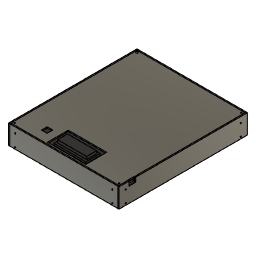
Case (Autodesk Fusion 360 design; units mm, degrees)
Autodesk Fusion 360 part; units mm, degrees
sketch "Sketch1" plane through (0, 0, 0) normal (0, 0, 1) x (1, 0, 0) in component "PCB"
  line L0 (-131, 153.5) -> (131, 153.5) construction
  line L1 (131, 153.5) -> (131, -153.5) construction
  line L2 (131, -153.5) -> (-131, -153.5) construction
  line L3 (-131, -153.5) -> (-131, 153.5) construction
  line L4 (-131, 153.5) -> (131, -153.5) construction
  line L5 (131, 153.5) -> (-131, -153.5) construction
  line L6 (-135, 157.5) -> (135, 157.5)
  line L7 (135, 157.5) -> (135, -157.5)
  line L8 (135, -157.5) -> (-135, -157.5)
  line L9 (-135, -157.5) -> (-135, 157.5)
  line L10 (-135, 157.5) -> (135, -157.5) construction
  line L11 (135, 157.5) -> (-135, -157.5) construction
  circle A0 centre (-131, 153.5) radius 1.6
  circle A1 centre (131, 153.5) radius 1.6
  circle A2 centre (-131, -153.5) radius 1.6
  circle A3 centre (131, -153.5) radius 1.6
  line L12 (135, -127.52) -> (128, -127.52) construction
  line L13 (128, -127.52) -> (128, -123.02)
  line L14 (128, -123.02) -> (135, -123.02)
  line L15 (128, -132.02) -> (135, -132.02)
  line L16 (128, -127.52) -> (128, -132.02)
  line L17 (122.64, -122.688) -> (112.36, -122.688)
  line L18 (112.36, -122.688) -> (112.36, -120.028)
  line L19 (112.36, -120.028) -> (122.64, -120.028)
  line L20 (122.64, -120.028) -> (122.64, -122.688)
  line L21 (122.64, -122.688) -> (112.36, -120.028) construction
  line L22 (112.36, -122.688) -> (122.64, -120.028) construction
  circle A4 centre (113.69, -121.358) radius 0.5
  circle A5 centre (116.23, -121.358) radius 0.5
  circle A6 centre (118.77, -121.358) radius 0.5
  circle A7 centre (121.31, -121.358) radius 0.5
  line L23 (113.69, -121.358) -> (116.23, -121.358) construction
  line L24 (116.23, -121.358) -> (118.77, -121.358) construction
  line L25 (118.77, -121.358) -> (121.31, -121.358) construction
  line L26 (121.31, -121.358) -> (122.64, -121.358) construction
  line L27 (113.69, -121.358) -> (112.36, -121.358) construction
  line L28 (-40.14, -109.718) -> (40.14, -109.718)
  line L29 (40.14, -109.718) -> (40.14, -145.998)
  line L30 (40.14, -145.998) -> (-40.14, -145.998)
  line L31 (-40.14, -145.998) -> (-40.14, -109.718)
  line L32 (-40.14, -109.718) -> (40.14, -145.998) construction
  line L33 (40.14, -109.718) -> (-40.14, -145.998) construction
  line L34 (-36.5, -115.358) -> (36.5, -115.358)
  line L35 (36.5, -115.358) -> (36.5, -140.358)
  line L36 (36.5, -140.358) -> (-36.5, -140.358)
  line L37 (-36.5, -140.358) -> (-36.5, -115.358)
  line L38 (-36.5, -115.358) -> (36.5, -140.358) construction
  line L39 (36.5, -115.358) -> (-36.5, -140.358) construction
  point P0 (117.5, -121.358)
  point P1 (0, -127.858)
  point P2 (0, -127.858)
  dimension "d1" = 262
  dimension "d2" = 307
  dimension "d3" = 270
  dimension "d4" = 315
  dimension "d5" = 3.2
  dimension "d8" = 29.98
  dimension "d9" = 9
  dimension "d10" = 7
  dimension "d17" = 10.28
  dimension "d18" = 2.66
  dimension "d19" = 2.54
  dimension "d20" = 1
  dimension "d21" = 36.142
  dimension "d22" = 17.5
  dimension "d30" = 29.642
  dimension "d31" = 135
  dimension "d32" = 80.28
  dimension "d33" = 36.28
  dimension "d34" = 73
  dimension "d35" = 25
  constraint horizontal L0
  constraint perpendicular L0 L1
  constraint parallel L0 L2
  constraint parallel L1 L3
  constraint coincident L4 origin
  constraint coincident L5 origin
  constraint horizontal L6
  constraint perpendicular L6 L7
  constraint parallel L6 L8
  constraint parallel L7 L9
  constraint coincident L10 origin
  constraint coincident L11 origin
  constraint coincident L0.start L3.end
  constraint coincident L0.end L1.start
  constraint coincident L2.end L3.start
  constraint coincident L1.end L2.start
  constraint equal A1 A3
  constraint equal A2 A3
  constraint equal A0 A2
  constraint coincident L7 L12.start
  constraint perpendicular L1 L12
  constraint perpendicular L12 L13
  constraint coincident L7 L14.end
  constraint perpendicular L7 L14
  constraint symmetric L13.start L12 L16.start
  constraint symmetric L12 L13.end L15.start
  constraint symmetric L12 L14.end L15.end
  constraint horizontal L17
  constraint perpendicular L17 L18
  constraint parallel L17 L19
  constraint parallel L18 L20
  constraint coincident L21 P0
  constraint coincident L22 P0
  constraint coincident A4.centre L23.start
  constraint horizontal L23
  constraint coincident A5.centre L23.end
  constraint equal A4 A5
  constraint equal A5 A6
  constraint equal A6 A7
  constraint parallel L23 L24
  constraint parallel L23 L25
  constraint parallel L25 L26
  constraint coincident A6.centre L24.end
  constraint coincident A7.centre L25.end
  constraint equal L23 L24
  constraint equal L24 L25
  constraint parallel L23 L27
  constraint equal L26 L27
  constraint midpoint L18 L27.end
  constraint midpoint L20 L26.end
  constraint horizontal L28
  constraint perpendicular L28 L29
  constraint parallel L28 L30
  constraint parallel L29 L31
  constraint coincident L32 P2
  constraint coincident L33 P2
  constraint horizontal L34
  constraint perpendicular L34 L35
  constraint parallel L34 L36
  constraint parallel L35 L37
  constraint coincident L38 P2
  constraint coincident L39 P2
  constraint coincident P2 P1
  measures "d1" distance of L1.end L2.end
  measures "d2" distance of L0.end L1.end
  measures "d3" distance of L7.end L8.end
  measures "d4" distance of L6.end L7.end
  measures "d5" diameter of A0
  measures "d8" distance of L7.end L12.start
  measures "d9" distance of L14 L15
  measures "d10" distance of L13.end L14.end
  measures "d17" distance of L18.end L19.end
  measures "d18" distance of L17.end L18.end
  measures "d19" distance of A4.centre A5.centre
  measures "d20" diameter of A7
  measures "d21" distance of L8 P0
  measures "d22" distance of L7 P0
  measures "d30" distance of L8 P2
  measures "d31" distance of L9 P2
  measures "d32" distance of L28.start L28.end
  measures "d33" distance of L28.end L29.end
  measures "d34" distance of L35.end L36.end
  measures "d35" distance of L34.end L35.end
extrude "Extrude1" add sketch "Sketch1" along normal blind 1.6 contours L6 L7 L8 L9 L13 L14 L15 L16 makes body 1 in component "PCB"
extrude "Extrude2" add sketch "Sketch1" along normal blind 5 contours L7 L13 L14 L15 L16 bodies 1 in component "PCB"
extrude "Extrude3" add sketch "Sketch1" along normal blind 6.2 contours L28 L29 L30 L31 bodies 1 in component "PCB"
extrude "Extrude4" add sketch "Sketch1" along normal blind 13.15 contours L34 L35 L36 L37 bodies 1 in component "PCB"
sketch "Sketch1 (2)" plane through (0, 0, 0) normal (0, 0, 1) x (1, 0, 0) in component "Corner"
  circle A0 centre (0, 0) radius 2.3
  line L0 (0, 0) -> (0, -9.2) construction
  line L1 (0, 0) -> (9.2, 0) construction
  circle A1 centre (0, -9.2) radius 2.3
  circle A2 centre (9.2, 0) radius 2.3
  line L2 (-4.6, 4.6) -> (-4.6, -13.8)
  line L3 (-4.6, -13.8) -> (4.6, -13.8)
  line L4 (4.6, -13.8) -> (4.6, -4.6)
  line L5 (4.6, -4.6) -> (13.8, -4.6)
  line L6 (13.8, -4.6) -> (13.8, 4.6)
  line L7 (13.8, 4.6) -> (-4.6, 4.6)
  line L8 (4.6, 0) -> (4.6, 4.6) construction
  line L9 (4.6, 0) -> (4.6, -4.6) construction
  line L10 (0, -4.6) -> (4.6, -4.6) construction
  line L11 (0, -4.6) -> (-4.6, -4.6) construction
  line L12 (9.2, 0) -> (13.8, 0) construction
  line L13 (0, -9.2) -> (0, -13.8) construction
  dimension "d41" = 4.6
  dimension "d42" = 9.2
  dimension "d43" = 4.6
  dimension "d44" = 4.6
  constraint coincident A0.centre L0.start
  constraint vertical L0
  constraint perpendicular L0 L1
  constraint equal L0 L1
  constraint coincident L0.end A1.centre
  constraint coincident L1.end A2.centre
  constraint equal A0 A2
  constraint equal A1 A2
  constraint vertical L2
  constraint perpendicular L2 L3
  constraint perpendicular L3 L4
  constraint perpendicular L4 L5
  constraint perpendicular L5 L6
  constraint perpendicular L6 L7
  constraint coincident L2.start L7.end
  constraint midpoint L1 L8.start
  constraint coincident L7 L8.end
  constraint perpendicular L7 L8
  constraint coincident L5 L4.end
  constraint perpendicular L5 L9
  constraint midpoint L0 L10.start
  constraint coincident L4 L5.start
  constraint perpendicular L4 L10
  constraint coincident L2 L11.end
  constraint perpendicular L2 L11
  constraint coincident L4.end L5.start
  constraint midpoint L6 L12.end
  constraint midpoint L3 L13.end
  constraint equal L11 L13
  constraint equal L12 L13
  measures "d41" diameter of A0
  measures "d42" distance of A0.centre L0.end
  measures "d43" distance of L8.start L8.end
  measures "d44" distance of L10.start L11.end
extrude "Extrude1'" add sketch "Sketch1 (2)" along normal blind 9 separate body contours A1 | A2 | L2 L3 L4 L5 L6 L7 makes body 2 in component "Corner"
extrude "Extrude2'" add sketch "Sketch1 (2)" along normal blind 3 contours A0 bodies 2 in component "Corner"
sketch "Sketch2" plane through (-4.6, 0, 0) normal (-1, 0, 0) x (0, -1, 0) in component "Corner"
  line L0 (-4.6, 0) -> (13.8, 0)
  line L1 (13.8, 0) -> (13.8, 9)
  line L2 (13.8, 9) -> (-4.6, 9)
  line L3 (-4.6, 9) -> (-4.6, 0)
  line L4 (11.5, 0) -> (6.9, 0)
  line L5 (13.8, 4.5) -> (9.2, 4.5) construction
  line L6 (9.2, 0) -> (9.2, 4.5) construction
  circle A0 centre (9.2, 4.5) radius 2.3
  dimension "d49" = 4.6
  constraint midpoint L1 L5.start
  constraint perpendicular L1 L5
  constraint midpoint L4 L6.start
  constraint perpendicular L4 L6
  constraint coincident L5.end L6.end
  measures "d49" diameter of A0
extrude "Extrude3'" cut sketch "Sketch2" against normal blind 6 contours A0 bodies 2 in component "Corner"
sketch "Sketch3" plane through (0, 4.6, 0) normal (0, 1, 0) x (-1, 0, 0) in component "Corner"
  line L0 (-13.8, 0) -> (4.6, 0)
  line L1 (4.6, 0) -> (4.6, 9)
  line L2 (4.6, 9) -> (-13.8, 9)
  line L3 (-13.8, 9) -> (-13.8, 0)
  line L4 (-6.9, 0) -> (-11.5, 0)
  line L5 (-13.8, 4.5) -> (-9.2, 4.5) construction
  line L6 (-9.2, 0) -> (-9.2, 4.5) construction
  circle A0 centre (-9.2, 4.5) radius 2.3
  dimension "d52" = 4.6
  constraint midpoint L3 L5.start
  constraint perpendicular L3 L5
  constraint midpoint L4 L6.start
  constraint perpendicular L4 L6
  constraint coincident L5.end L6.end
  measures "d52" diameter of A0
extrude "Extrude4'" cut sketch "Sketch3" against normal blind 6 contours A0 bodies 2 in component "Corner"
sketch "Sketch1 (3)" plane through (0, 0, 0) normal (0, 0, 1) x (1, 0, 0) in component "Washer"
  circle A0 centre (0, 0) radius 1.6
  circle A1 centre (0, 0) radius 2.6
  dimension "d55" = 3.2
  dimension "d56" = 1
  constraint coincident A0.centre A1.centre
  measures "d55" diameter of A0
extrude "Extrude1''" add sketch "Sketch1 (3)" along normal blind 1 separate body makes body 3 in component "Washer"
sketch "Sketch1 (4)" plane through (0, 0, 0) normal (0, 0, 1) x (1, 0, 0) in component "PlateWasher"
  circle A0 centre (0, 0) radius 1.6
  circle A1 centre (0, 0) radius 2.6
  dimension "d59" = 3.2
  dimension "d60" = 1
  constraint coincident A0.centre A1.centre
  measures "d59" diameter of A0
extrude "Extrude1'''" add sketch "Sketch1 (4)" along normal blind 4 separate body makes body 4 in component "PlateWasher"
move_face "OffsetFaces1" offset 30 1 faces at (4.6, 1.5333, 0) on bodies 2 in component "Corner"
sketch "Sketch5" plane through (0, 4.6, 0) normal (0, 1, 0) x (-1, 0, 0) in component "Corner"
  circle A0 centre (-9.2, 4.5) radius 2.3
  line L0 (-13.8, -30) -> (4.6, -30)
  line L1 (4.6, -30) -> (4.6, 9)
  line L2 (4.6, 9) -> (-13.8, 9)
  line L3 (-13.8, 9) -> (-13.8, -30)
  line L4 (-9.2, 4.5) -> (-9.2, 9) construction
  line L5 (-9.2, -30) -> (-9.2, -25.5) construction
  circle A1 centre (-9.2, -25.5) radius 2.3
  line L6 (-9.2, -25.5) -> (-9.2, 4.5) construction
  constraint coincident A0.centre L4.start
  constraint coincident L2 L4.end
  constraint perpendicular L2 L4
  constraint coincident L0 L5.start
  constraint perpendicular L0 L5
  constraint coincident L5.end A1.centre
  constraint equal A0 A1
  constraint equal L4 L5
  constraint vertical L6
extrude "Extrude6" cut sketch "Sketch5" against normal up to surface (6 mm away) contours A1 bodies 2 in component "Corner"
sketch "Sketch6" plane through (-4.6, 0, 0) normal (-1, 0, 0) x (0, -1, 0) in component "Corner"
  circle A0 centre (9.2, 4.5) radius 2.3
  line L0 (-4.6, -30) -> (13.8, -30)
  line L1 (13.8, -30) -> (13.8, 9)
  line L2 (13.8, 9) -> (-4.6, 9)
  line L3 (-4.6, 9) -> (-4.6, -30)
  line L4 (9.2, 4.5) -> (9.2, 9) construction
  line L5 (9.2, -30) -> (9.2, -25.5) construction
  line L6 (9.2, -25.5) -> (9.2, 4.5) construction
  circle A1 centre (9.2, -25.5) radius 2.3
  constraint coincident A0.centre L4.start
  constraint coincident L2 L4.end
  constraint perpendicular L2 L4
  constraint coincident L0 L5.start
  constraint perpendicular L0 L5
  constraint parallel L4 L6
  constraint equal L4 L5
  constraint coincident L5.end L6.start
  constraint equal A0 A1
extrude "Extrude7" cut sketch "Sketch6" against normal up to surface (6 mm away) contours A1 bodies 2 in component "Corner"
sketch "Sketch1 (5)" plane through (0, -158.1, 0) normal (0, -1, 0) x (1, 0, 0) in component "Panel1"
  circle A0 centre (-121.8, -35.5) radius 2.3
  circle A1 centre (-121.8, -5.5) radius 2.3
  line L0 (-135.6, -40) -> (-117.2, -40)
  line L1 (-117.2, -40) -> (-117.2, -1)
  line L2 (-117.2, -1) -> (-135.6, -1)
  line L3 (-135.6, -1) -> (-135.6, -40)
  circle A2 centre (121.8, -35.5) radius 2.3
  circle A3 centre (121.8, -5.5) radius 2.3
  line L4 (117.2, -40) -> (135.6, -40)
  line L5 (135.6, -40) -> (135.6, -1)
  line L6 (135.6, -1) -> (117.2, -1)
  line L7 (117.2, -1) -> (117.2, -40)
  line L8 (-117.2, -40) -> (117.2, -40)
  line L9 (-128.4, 5.6) -> (-133.6, 5.6)
  line L10 (-135.6, -1) -> (-135.6, 5.6)
  line L11 (-135.6, 5.6) -> (-133.6, 5.6) construction
  line L12 (-135.6, 5.6) -> (-135.6, 8.6)
  line L13 (135.6, -1) -> (135.6, 8.6)
  line L14 (135.6, 8.6) -> (-135.6, 8.6)
  circle A4 centre (-121.8, -5.5) radius 1.6
  circle A5 centre (-121.8, -35.5) radius 1.6
  circle A6 centre (121.8, -5.5) radius 1.6
  circle A7 centre (121.8, -35.5) radius 1.6
  dimension "d120" = 3
  dimension "d123" = 3.2
  constraint coincident L0.end L1.start
  constraint coincident L4.start L7.end
  constraint coincident L2.end L3.start
  constraint perpendicular L2 L10
  constraint coincident L9.end L11.end
  constraint perpendicular L10 L11
  constraint perpendicular L11 L12
  constraint coincident L5.end L6.start
  constraint perpendicular L6 L13
  constraint perpendicular L12 L14
  constraint concentric A1 A4
  constraint concentric A0 A5
  constraint concentric A3 A6
  constraint concentric A2 A7
  constraint equal A6 A7
  constraint equal A4 A6
  constraint equal A4 A5
  measures "d120" distance of L10.end L12.end
  measures "d123" diameter of A4
extrude "Extrude1''''" add sketch "Sketch1 (5)" along normal blind 3 separate body contours A0 | A1 | L0 L1 L2 L3 | L1 L2 L6 L7 L8 L10 L12 L13 L14 | L4 L5 L6 L7 | A2 | A3 makes body 5 in component "Panel1"
sketch "Sketch1 (6)" plane through (135.6, 0, 0) normal (1, 0, 0) x (0, 1, 0) in component "Panel2"
  circle A0 centre (-144.3, -35.5) radius 2.3
  circle A1 centre (-144.3, -5.5) radius 2.3
  line L0 (-158.1, -40) -> (-139.7, -40)
  line L1 (-139.7, -40) -> (-139.7, -1)
  line L2 (-139.7, -1) -> (-158.1, -1)
  line L3 (-158.1, -1) -> (-158.1, -40)
  circle A2 centre (144.3, -35.5) radius 2.3
  circle A3 centre (144.3, -5.5) radius 2.3
  line L4 (139.7, -40) -> (158.1, -40)
  line L5 (158.1, -40) -> (158.1, -1)
  line L6 (158.1, -1) -> (139.7, -1)
  line L7 (139.7, -1) -> (139.7, -40)
  line L8 (-158.1, -40) -> (-158.1, 8.6)
  line L9 (-158.1, 8.6) -> (-161.1, 8.6)
  line L10 (-161.1, 8.6) -> (-161.1, -40)
  line L11 (-161.1, -40) -> (-158.1, -40)
  line L12 (161.1, -40) -> (161.1, 8.6)
  line L13 (161.1, 8.6) -> (158.1, 8.6)
  line L14 (158.1, 8.6) -> (158.1, -40)
  line L15 (158.1, -40) -> (161.1, -40)
  line L16 (139.7, -40) -> (-139.7, -40)
  line L17 (-158.1, 8.6) -> (158.1, 8.6)
  line L18 (-157.5, 0) -> (157.5, 0)
  line L19 (157.5, 0) -> (157.5, 1.6)
  line L20 (157.5, 1.6) -> (-123.02, 1.6)
  line L21 (-123.02, 1.6) -> (-123.02, 5)
  line L22 (-123.02, 5) -> (-132.02, 5)
  line L23 (-132.02, 5) -> (-132.02, 1.6)
  line L24 (-132.02, 1.6) -> (-157.5, 1.6)
  line L25 (-157.5, 1.6) -> (-157.5, 0)
  line L26 (-132.02, 5) -> (-123.02, 5) construction
  line L27 (-123.02, 5) -> (-123.02, 1.6) construction
  line L28 (-123.02, 1.6) -> (-132.02, 1.6) construction
  line L29 (-132.02, 1.6) -> (-132.02, 5) construction
  line L30 (-136.02, 9) -> (-119.02, 9)
  line L31 (-119.02, 9) -> (-119.02, -2.4)
  line L32 (-119.02, -2.4) -> (-136.02, -2.4)
  line L33 (-136.02, -2.4) -> (-136.02, 9)
  circle A4 centre (-144.3, -5.5) radius 1.6
  circle A5 centre (-144.3, -35.5) radius 1.6
  circle A6 centre (144.3, -5.5) radius 1.6
  circle A7 centre (144.3, -35.5) radius 1.6
  dimension "d128" = -4
  dimension "d129" = 3.2
  constraint coincident L4.start L7.end
  constraint coincident L0.end L1.start
  constraint coincident L8.end L9.start
  constraint coincident L13.end L14.start
  constraint horizontal L26
  constraint vertical L27
  constraint horizontal L28
  constraint vertical L29
  constraint coincident L20.end L21.start
  constraint coincident L22.end L23.start
  constraint concentric A1 A4
  constraint concentric A0 A5
  constraint concentric A3 A6
  constraint concentric A2 A7
  constraint equal A6 A7
  constraint equal A4 A6
  constraint equal A4 A5
  measures "d129" diameter of A5
extrude "Extrude1'''''" add sketch "Sketch1 (6)" along normal blind 3 separate body contours A0 | A1 | L0 L1 L2 L3 L8 | L3 L8 L9 L10 L11 | L1 L2 L6 L7 L8 L14 L16 L17 L18 L19 L20 L24 L25 L31 L32 L33 | L4 L5 L6 L7 L14 | L5 L12 L13 L14 L15 | L18 L24 L25 L33 | L18 L19 L20 L31 | A2 | A3 makes body 6 in component "Panel2"
sketch "Sketch1 (7)" plane through (-135.6, 0, 0) normal (-1, 0, 0) x (0, -1, 0) in component "Panel3"
  circle A0 centre (-144.3, -35.5) radius 2.3
  circle A1 centre (-144.3, -5.5) radius 2.3
  line L0 (-158.1, -40) -> (-139.7, -40)
  line L1 (-139.7, -40) -> (-139.7, -1)
  line L2 (-139.7, -1) -> (-158.1, -1)
  line L3 (-158.1, -1) -> (-158.1, -40)
  circle A2 centre (-144.3, -35.5) radius 1.6
  circle A3 centre (-144.3, -5.5) radius 1.6
  circle A4 centre (144.3, -35.5) radius 1.6
  circle A5 centre (144.3, -5.5) radius 1.6
  line L4 (119.02, -2.4) -> (119.02, 8.6)
  line L5 (119.02, 8.6) -> (-161.1, 8.6)
  line L6 (-161.1, 8.6) -> (-161.1, -40)
  line L7 (-161.1, -40) -> (161.1, -40)
  line L8 (161.1, -40) -> (161.1, 8.6)
  line L9 (161.1, 8.6) -> (136.02, 8.6)
  line L10 (136.02, 8.6) -> (136.02, -2.4)
  line L11 (136.02, -2.4) -> (119.02, -2.4)
  line L12 (136.02, 8.6) -> (119.02, 8.6)
  constraint coincident L9.end L10.start
  constraint coincident L4.end L5.start
extrude "Extrude1''''''" add sketch "Sketch1 (7)" along normal blind 3 separate body contours A0 | A1 | L0 L1 L2 L3 L7 | L1 L2 L3 L4 L5 L6 L7 L8 L9 L10 L11 | L4 L10 L11 L12 makes body 7 in component "Panel3"
sketch "Sketch1 (8)" plane through (0, 0, 5.6) normal (0, 0, 1) x (-1, 0, 0) in component "TopPanel"
  circle A0 centre (131, -153.5) radius 1.6
  circle A1 centre (131, -153.5) radius 2.6
  circle A2 centre (131, -153.5) radius 1.6
  circle A3 centre (-131, -153.5) radius 1.6
  circle A4 centre (-131, 153.5) radius 1.6
  circle A5 centre (131, 153.5) radius 1.6
  line L0 (135.6, 161.1) -> (135.6, -161.1)
  line L1 (135.6, -161.1) -> (138.6, -161.1)
  line L2 (138.6, -161.1) -> (138.6, 161.1)
  line L3 (138.6, 161.1) -> (135.6, 161.1)
  line L4 (-135.6, 158.1) -> (135.6, 158.1)
  line L5 (135.6, 158.1) -> (135.6, 161.1)
  line L6 (135.6, 161.1) -> (-135.6, 161.1)
  line L7 (-135.6, 161.1) -> (-135.6, 158.1)
  line L8 (-135.6, 136.02) -> (-135.6, 161.1)
  line L9 (-135.6, 161.1) -> (-138.6, 161.1)
  line L10 (-138.6, 161.1) -> (-138.6, 136.02)
  line L11 (-138.6, 136.02) -> (-135.6, 136.02)
  line L12 (-135.6, 119.02) -> (-135.6, 136.02)
  line L13 (-135.6, 136.02) -> (-138.6, 136.02)
  line L14 (-138.6, 136.02) -> (-138.6, 119.02)
  line L15 (-138.6, 119.02) -> (-135.6, 119.02)
  line L16 (-135.6, -161.1) -> (-135.6, 119.02)
  line L17 (-135.6, 119.02) -> (-138.6, 119.02)
  line L18 (-138.6, 119.02) -> (-138.6, -161.1)
  line L19 (-138.6, -161.1) -> (-135.6, -161.1)
  line L20 (-135.6, -161.1) -> (135.6, -161.1)
  line L21 (135.6, -161.1) -> (135.6, -158.1)
  line L22 (135.6, -158.1) -> (-135.6, -158.1)
  line L23 (-135.6, -158.1) -> (-135.6, -161.1)
  line L24 (-112.36, 120.028) -> (-122.64, 120.028)
  line L25 (-122.64, 120.028) -> (-122.64, 122.688)
  line L26 (-122.64, 122.688) -> (-112.36, 122.688)
  line L27 (-112.36, 122.688) -> (-112.36, 120.028)
  circle A6 centre (131, -153.5) radius 1.6
  circle A7 centre (-131, 153.5) radius 1.6
  circle A8 centre (131, 153.5) radius 1.6
  circle A9 centre (-131, -153.5) radius 1.6
  line L28 (-40.14, 145.998) -> (40.14, 145.998)
  line L29 (40.14, 145.998) -> (40.14, 109.718)
  line L30 (40.14, 109.718) -> (-40.14, 109.718)
  line L31 (-40.14, 109.718) -> (-40.14, 145.998)
  line L32 (-128, 123.02) -> (-135, 123.02)
  line L33 (-135, 123.02) -> (-135, -157.5)
  line L34 (-135, -157.5) -> (135, -157.5)
  line L35 (135, -157.5) -> (135, 157.5)
  line L36 (135, 157.5) -> (-135, 157.5)
  line L37 (-135, 157.5) -> (-135, 132.02)
  line L38 (-135, 132.02) -> (-128, 132.02)
  line L39 (-128, 132.02) -> (-128, 123.02)
  line L40 (-135.6, 136.02) -> (-135, 136.02)
  line L41 (-135.6, 119.02) -> (-135, 119.02)
  line L42 (-135, 123.02) -> (-135, 132.02)
  line L43 (-48.14, 153.998) -> (48.14, 153.998)
  line L44 (48.14, 153.998) -> (48.14, 101.718)
  line L45 (48.14, 101.718) -> (-48.14, 101.718)
  line L46 (-48.14, 101.718) -> (-48.14, 153.998)
  line L47 (82.025, 120.833) -> (67.975, 120.833)
  line L48 (67.975, 120.833) -> (67.975, 134.883)
  line L49 (67.975, 134.883) -> (82.025, 134.883)
  line L50 (82.025, 134.883) -> (82.025, 120.833)
  line L51 (82.025, 120.833) -> (67.975, 134.883) construction
  line L52 (67.975, 120.833) -> (82.025, 134.883) construction
  point P0 (75, 127.858)
  dimension "d136" = -8
  dimension "d138" = 14.05
  dimension "d139" = 60
  dimension "d140" = 29.642
  constraint coincident L8.start L11.end
  constraint coincident L37 L40.end
  constraint perpendicular L37 L40
  constraint coincident L12.start L15.end
  constraint coincident L33 L41.end
  constraint perpendicular L33 L41
  constraint coincident L32.end L33.start
  constraint coincident L37.end L38.start
  constraint horizontal L47
  constraint perpendicular L47 L48
  constraint parallel L47 L49
  constraint parallel L48 L50
  constraint coincident L51 P0
  constraint coincident L52 P0
  constraint equal L48 L49
  measures "d138" distance of L47.end L48.end
  measures "d139" distance of L35 P0
  measures "d140" distance of L36 P0
extrude "Extrude1'''''''" add sketch "Sketch1 (8)" along normal blind 3 separate body contours L0 L4 L8 L16 L22 L33 L34 L35 L36 L37 L40 L41 | L32 L33 L34 L35 L36 L37 L38 L39 | L32 L38 L39 L42 | L24 L25 L26 L27 makes body 8 in component "TopPanel"
component "PCB" placed x (1, 0, 0) y (0, 1, 0) z (0, 0, 1) at (0, 0, 0)
component "Connectors" placed x (1, 0, 0) y (0, 1, 0) z (0, 0, 1) at (0, 0, 0)
component "Hardware" placed x (1, 0, 0) y (0, 1, 0) z (0, 0, 1) at (0, 0, 0)
component "Panels" placed x (1, 0, 0) y (0, 1, 0) z (0, 0, 1) at (0, 0, 0)
component "Corner" placed x (1, 0, 0) y (0, 1, 0) z (0, 0, 1) at (-131, 153.5, -10) in component "Connectors"
component "Washer" placed x (0, -1, 0) y (1, 0, 0) z (0, 0, 1) at (131, 153.5, -1) in component "Connectors"
component "PlateWasher" placed x (1, 0, 0) y (0, 1, 0) z (0, 0, 1) at (-131, -153.5, 1.6) in component "Connectors"
component "Corner" placed x (0, -1, 0) y (1, 0, 0) z (0, 0, 1) at (131, 153.5, -10) in component "Connectors"
component "Corner" placed x (-1, 0, 0) y (0, -1, 0) z (0, 0, 1) at (131, -153.5, -10) in component "Connectors"
component "Corner" placed x (0, 1, 0) y (-1, 0, 0) z (0, 0, 1) at (-131, -153.5, -10) in component "Connectors"
component "Washer" placed x (0, 1, 0) y (-1, 0, 0) z (0, 0, 1) at (-131, -153.5, -1) in component "Connectors"
component "Washer" placed x (1, 0, 0) y (0, 1, 0) z (0, 0, 1) at (-131, 153.5, -1) in component "Connectors"
component "Washer" placed x (-1, 0, 0) y (0, -1, 0) z (0, 0, 1) at (131, -153.5, -1) in component "Connectors"
component "PlateWasher" placed x (1, 0, 0) y (0, 1, 0) z (0, 0, 1) at (131, 153.5, 1.6) in component "Connectors"
component "PlateWasher" placed x (1, 0, 0) y (0, 1, 0) z (0, 0, 1) at (-131, 153.5, 1.6) in component "Connectors"
component "PlateWasher" placed x (1, 0, 0) y (0, 1, 0) z (0, 0, 1) at (131, -153.5, 1.6) in component "Connectors"
component "Panel1" placed x (1, 0, 0) y (0, 1, 0) z (0, 0, 1) at (0, 319.2, 0) in component "Panels"
component "Panel1" placed x (1, 0, 0) y (0, 1, 0) z (0, 0, 1) at (0, 0, 0) in component "Panels"
component "Panel2" placed x (1, 0, 0) y (0, 1, 0) z (0, 0, 1) at (0, 0, 0) in component "Panels"
component "Panel3" placed x (1, 0, 0) y (0, 1, 0) z (0, 0, 1) at (0, 0, 0) in component "Panels"
component "TopPanel" placed x (1, 0, 0) y (0, 1, 0) z (0, 0, 1) at (0, 0, 0) in component "Panels"
equation "BoltHoleDiameter = 3.2 mm"
equation "HeatInsertDiameter = 4.6 mm"
equation "HeatInsertLength = 6 mm"
equation "PCBToPlate = 4 mm" comment "Distance from top of PCB to the bottom of plate"
equation "MaterialThickness = 3 mm" comment "Laser cut material thickness"
equation "d36 = 1.6 mm + 3 mm + 1.6 mm"
equation "WasherThickness = 1 mm" comment "Must be multiple of PCBToPlate"
equation "d41 = HeatInsertDiameter"
equation "d42 = HeatInsertDiameter * 2"
equation "d43 = HeatInsertDiameter"
equation "d44 = HeatInsertDiameter"
equation "d45 = HeatInsertLength + 3 mm"
equation "d49 = HeatInsertDiameter"
equation "d50 = -HeatInsertLength"
equation "d52 = HeatInsertDiameter"
equation "d53 = -HeatInsertLength"
equation "d55 = BoltHoleDiameter"
equation "d57 = WasherThickness"
equation "d59 = BoltHoleDiameter"
equation "d61 = PCBToPlate"
equation "d120 = MaterialThickness"
equation "d121 = MaterialThickness"
equation "d123 = BoltHoleDiameter"
equation "d129 = BoltHoleDiameter"
equation "d130 = MaterialThickness"
equation "d132 = MaterialThickness"
equation "d134 = MaterialThickness"
